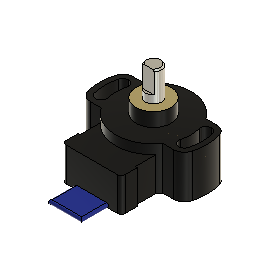
Gas Pedal Sensor Adapter (Autodesk Fusion 360 archive; units mm, degrees)
design "Rotary Hall Effect Pedal Sensor PSC360G2-F2AA-C0002-ERA360-05K"
Autodesk Fusion 360 part; units mm, degrees
note: some values were not read from the file. Chosen so that the rebuilt part matches the saved one: which face or edge a step refers to; that a step has no effect. Set by a fixed rule: which sketch regions a step uses.
sketch "Sketch1" plane through (0, 0, 0) normal (0, 0, 1) x (1, 0, 0)
  circle A0 centre (0, 0) radius 16 construction
  circle A1 centre (0, 0) radius 14
  dimension "d1" = 32
  dimension "d2" = 28
  constraint coincident A0.centre A1.centre
  measures "d1" diameter of A0
  measures "d2" diameter of A1
extrude "Extrude1" add sketch "Sketch1" along normal blind 16
sketch "Sketch2" plane through (0, 0, 0) normal (0, 0, 1) x (1, 0, 0)
  line L0 (0, 0) -> (0, -17) construction
  circle A0 centre (0, 0) radius 14 construction
  line L1 (0, 14) -> (0, -23) construction
  line L2 (0, -23) -> (-11, -23) construction
  line L3 (-11, -23) -> (11, -23)
  line L4 (11, -23) -> (11, -17)
  line L5 (11, -6.2827) -> (-11, -6.2827)
  line L6 (-10.3, -17) -> (-11, -17)
  line L7 (-10.3, -17) -> (-10.3, -4.6882)
  line L8 (-11, -6.2827) -> (-11, -8.6603)
  line L9 (-11, -17) -> (-11, -23)
  line L10 (0, -17) -> (10.3, -17) construction
  line L11 (10.3, -17) -> (11, -17)
  line L12 (10.3, -17) -> (10.3, -1.724)
  dimension "d5" = 17
  dimension "d6" = 37
  dimension "d7" = 11
  dimension "d8" = 22
  dimension "d9" = 10.3
  dimension "d10" = 10.3
  constraint coincident L0.start A0.centre
  constraint vertical L0
  constraint coincident A0 L1.start
  constraint parallel L0 L1
  constraint perpendicular L1 L2
  constraint horizontal L3
  constraint vertical L4
  constraint horizontal L5
  constraint vertical L8
  constraint coincident L6.end L8
  constraint perpendicular L6 L8
  constraint perpendicular L5 L7
  constraint coincident A0 L8.end
  constraint collinear L8 L9
  constraint perpendicular L4 L10
  constraint perpendicular L4 L11
  constraint perpendicular L5 L12
  measures "d5" distance of L0.start L0.end
  measures "d6" distance of L1.start L1.end
  measures "d7" distance of L1.end L2.end
  measures "d8" distance of L2.end L3.end
  measures "d9" distance of L0.end L6.start
  measures "d10" distance of L0.end L10.end
extrude "Extrude2" add sketch "Sketch2" along normal blind 12.5
sketch "Sketch3" plane through (0, 0, 0) normal (0, 0, 1) x (1, 0, 0)
  circle A0 centre (0, 0) radius 20
  line L0 (26.1704, -8) -> (-26.1704, -8)
  line L1 (-26.1704, -8) -> (-26.1704, 8)
  line L2 (-26.1704, 8) -> (26.1704, 8)
  line L3 (26.1704, 8) -> (26.1704, -8)
  line L4 (26.1704, -8) -> (-26.1704, 8) construction
  line L5 (-26.1704, -8) -> (26.1704, 8) construction
  dimension "d13" = 40
  dimension "d14" = 16
  constraint coincident A0.centre origin
  constraint horizontal L0
  constraint perpendicular L0 L1
  constraint parallel L0 L2
  constraint parallel L1 L3
  constraint coincident L4 A0.centre
  constraint coincident L5 A0.centre
  measures "d13" diameter of A0
  measures "d14" distance of L0.end L1.end
extrude "Extrude3" add sketch "Sketch3" along normal blind 16 contours A0 L0 L2
sketch "Sketch4" plane through (0, 0, 0) normal (0, 0, 1) x (1, 0, 0)
  circle A0 centre (-16, 0) radius 2.1
  circle A1 centre (0, 0) radius 16
  circle A2 centre (16, 0) radius 2.1
  circle A3 centre (0, 0) radius 14
  dimension "d17" = 4.2
  dimension "d18" = 4.2
  dimension "d19" = 28
  constraint coincident A0.centre A1
  constraint coincident A1 A2.centre
  constraint concentric A1 A3
  measures "d17" diameter of A0
  measures "d18" diameter of A2
  measures "d19" diameter of A3
extrude "Extrude4" cut sketch "Sketch4" along normal blind 50 contours A0 A3 | A0 A1 A3 | A0 A1 | A2 A3 | A1 A2 A3 | A1 A2
sketch "Sketch5" plane through (0, 0, 16) normal (0, 0, 1) x (-1, 0, 0)
  circle A0 centre (16, 0) radius 2.1
  circle A1 centre (-16, 0) radius 2.1
  arc A2 (11.4891, 8) -> (-11.4891, 8) centre (0, 0) ccw
  line L0 (-11.4891, 8) -> (-18.3303, 8)
  arc A3 (-18.3303, 8) -> (-18.3303, -8) centre (0, 0) ccw
  line L1 (-18.3303, -8) -> (-11.4891, -8)
  arc A4 (-11.4891, -8) -> (11.4891, -8) centre (0, 0) ccw
  line L2 (11.4891, -8) -> (18.3303, -8)
  arc A5 (18.3303, -8) -> (18.3303, 8) centre (0, 0) ccw
  line L3 (18.3303, 8) -> (11.4891, 8)
  line L4 (17.0411, 6.1) -> (10.4499, 6.1)
  arc A6 (10.4499, 6.1) -> (-10.4499, 6.1) centre (0, 0) ccw
  line L5 (-10.4499, 6.1) -> (-17.0411, 6.1)
  arc A7 (-17.0411, 6.1) -> (-17.0411, -6.1) centre (0, 0) ccw
  line L6 (-17.0411, -6.1) -> (-10.4499, -6.1)
  arc A8 (-10.4499, -6.1) -> (10.4499, -6.1) centre (0, 0) ccw
  line L7 (10.4499, -6.1) -> (17.0411, -6.1)
  arc A9 (17.0411, -6.1) -> (17.0411, 6.1) centre (0, 0) ccw
  circle A10 centre (15.4915, -4) radius 2.1
  dimension "d22" = -1.9
  dimension "d23" = 4.2
  dimension "d24" = 2.1
  measures "d23" diameter of A10
  measures "d24" distance of L7 A10.centre
ref_plane "WorkPlane1" through (-14.9097, 0, 8) normal (0, -1, 0) x (1, 0, 0)
extrude "Extrude5" cut sketch "Sketch5" against normal blind 20.219 contours A0 A10 | A0 A10 picked at (15.8466, -1.9917) picked at (15.4687, -4.7533)
mirror "Mirror1" about plane through (-14.9097, 0, 8) normal (0, -1, 0) of "Extrude5"
sketch "Sketch6" plane through (0, 0, 16) normal (0, 0, 1) x (-1, 0, 0)
  arc A0 (16.3288, 2.0741) -> (15.1628, 1.9259) centre (15.4915, 4) ccw
  arc A1 (16.3288, -2.0741) -> (16.3288, 2.0741) centre (16, 0) ccw
  arc A2 (15.1628, -1.9259) -> (16.3288, -2.0741) centre (15.4915, -4) ccw
  arc A3 (15.1628, 1.9259) -> (15.1628, -1.9259) centre (16, 0) ccw
  circle A4 centre (-16, 0) radius 2.1
  arc A5 (11.4891, 8) -> (-11.4891, 8) centre (0, 0) ccw
  line L0 (-11.4891, 8) -> (-18.3303, 8)
  arc A6 (-18.3303, 8) -> (-18.3303, -8) centre (0, 0) ccw
  line L1 (-18.3303, -8) -> (-11.4891, -8)
  arc A7 (-11.4891, -8) -> (11.4891, -8) centre (0, 0) ccw
  line L2 (11.4891, -8) -> (18.3303, -8)
  arc A8 (18.3303, -8) -> (18.3303, 8) centre (0, 0) ccw
  line L3 (18.3303, 8) -> (11.4891, 8)
  circle A9 centre (0, 0) radius 18.0935
  line L4 (17.0402, 6.0832) -> (11.3307, 6.0832)
  line L5 (15.4915, -4) -> (15.5034, -6.1)
  line L6 (17.4872, -6.0832) -> (10.4705, -6.123)
  circle A10 centre (0, 0) radius 13.9
  dimension "d30" = 90
  constraint concentric A5 A9
  constraint coincident A9 L4.start
  constraint horizontal L4
  constraint coincident A2.centre L5.start
  constraint coincident A2 L5.end
  constraint concentric A9 A10
  constraint tangent A3 A10
  measures "d30" angle of L5 L6
extrude "Extrude6" cut sketch "Sketch6" against normal blind 50 contours A0 A1 A9 | A0 A9 L4 | A1 A2 A9 | A0 L4 A10 | A2 A9 L6 | A0 A3 A10 | A2 A3 A10 | A2 L6 A10
delete_face "DeleteFace1" 1 faces at (-17.5465, 4.4327, 10.6667)
delete_face "DeleteFace2" 1 faces at (-15.3853, 6.0973, 10.6667)
delete_face "DeleteFace3" 1 faces at (-18.0955, 0.1367, 10.6667)
delete_face "DeleteFace4" 1 faces at (-15.3442, -6.0948, 5.3333)
delete_face "DeleteFace5" 1 faces at (-17.5295, -4.5066, 10.6667)
delete_face "DeleteFace6" 1 faces at (-15.5262, -6.0832, 10.6667)
fillet "Fillet1" radius 2.1 4 edges at (-17.0393, 6.0858, 8) (-12.4843, 6.1116, 8) (-12.4982, -6.0832, 8) (-17.0402, -6.0832, 8)
delete_face "DeleteFace7" [no effect]
mirror "Mirror2" about plane through (0, 0, 0) normal (1, 0, 0) of 6 faces at (-17.4233, -4.805, 10.6667) (-18.03, -1.515, 10.6667) (-14.2896, -5.7091, 10.6667) (-13.7624, 1.9509, 5.3333) (-15.1741, 6.0721, 10.6667) (-17.2821, 5.0874, 10.6667)
delete_face "DeleteFace8" 1 faces at (18.0955, 0.1367, 10.6667)
sketch "Sketch7" plane through (0, 0, 16) normal (0, 0, 1) x (-1, 0, 0)
  arc A0 (-17.4755, 4.6884) -> (-17.5201, -4.519) centre (0, 0) ccw
  arc A1 (-15.4974, 6.0832) -> (-17.4755, 4.6884) centre (-15.4974, 3.9832) ccw
  line L0 (-15.4974, 6.0832) -> (-15.4963, 6.0832)
  arc A2 (-13.4624, 3.4604) -> (-15.4963, 6.0832) centre (-15.4963, 3.9832) ccw
  arc A3 (-13.4624, 3.4604) -> (-13.4598, -3.4702) centre (0, 0) ccw
  arc A4 (-15.4985, -6.0945) -> (-13.4598, -3.4702) centre (-15.4934, -3.9945) ccw
  arc A5 (-17.5201, -4.519) -> (-15.4985, -6.0945) centre (-15.4866, -3.9945) ccw
  arc A6 (18.3303, -8) -> (18.3303, 8) centre (0, 0) ccw
  line L1 (18.3303, 8) -> (11.4891, 8)
  arc A7 (11.4891, 8) -> (-11.4891, 8) centre (0, 0) ccw
  line L2 (-11.4891, 8) -> (-18.3303, 8)
  arc A8 (-18.3303, 8) -> (-18.3303, -8) centre (0, 0) ccw
  line L3 (-18.3303, -8) -> (-11.4891, -8)
  arc A9 (-11.4891, -8) -> (11.4891, -8) centre (0, 0) ccw
  line L4 (11.4891, -8) -> (18.3303, -8)
  arc A10 (17.4755, 4.6884) -> (15.4974, 6.0832) centre (15.4974, 3.9832) ccw
  arc A11 (17.5201, -4.519) -> (17.4755, 4.6884) centre (0, 0) ccw
  arc A12 (15.4985, -6.0945) -> (17.5201, -4.519) centre (15.4866, -3.9945) ccw
  arc A13 (13.4598, -3.4702) -> (15.4985, -6.0945) centre (15.4934, -3.9945) ccw
  arc A14 (13.4598, -3.4702) -> (13.4624, 3.4604) centre (0, 0) ccw
  arc A15 (15.4963, 6.0832) -> (13.4624, 3.4604) centre (15.4963, 3.9832) ccw
  line L5 (15.4963, 6.0832) -> (15.4974, 6.0832)
  circle A16 centre (0, 0) radius 6.5
  dimension "d37" = 13
  constraint concentric A0 A16
  measures "d37" diameter of A16
extrude "Extrude7" add sketch "Sketch7" along normal blind 5.1 contours A16
sketch "Sketch8" plane through (0, 0, 21.1) normal (0, 0, 1) x (-1, 0, 0)
  circle A0 centre (0, 0) radius 6.5
  circle A1 centre (0, 0) radius 3
  dimension "d40" = 6
  constraint coincident A0.centre A1.centre
  measures "d40" diameter of A1
extrude "Extrude8" add sketch "Sketch8" along normal blind 9.9 contours A1
sketch "Sketch9" plane through (0, 0, 31) normal (0, 0, 1) x (-1, 0, 0)
  circle A0 centre (0, 0) radius 3
  line L0 (0, 0) -> (0.0009, -3) construction
  line L1 (0.0009, -3) -> (-0.0006, 2) construction
  line L2 (3.0076, 2) -> (-4.3795, 1.9979) construction
  line L3 (2.2363, 1.9998) -> (-3.6797, 1.9981)
  dimension "d43" = 5
  constraint coincident A0.centre L0.start
  constraint coincident A0 L0.end
  constraint parallel L0 L1
  constraint perpendicular L1 L2
  constraint coincident L2 L3.start
  constraint coincident A0 L3.start
  constraint coincident L2 L3.end
  constraint perpendicular L1 L3
  measures "d43" distance of L0.end L1.end
extrude "Extrude9" cut sketch "Sketch9" against normal blind 8 contours A0 L3 picked at (0.0625, 2.4741)
extrude "Extrude10" add 1 faces at (-0.7146, 0.4907, 31) along direction (0, 0, 1) blind 1
extrude "Extrude11" add 1 faces at (-0.0625, -2.4741, 23) along direction (0, 0, 1) blind 1
chamfer "Chamfer1" distance 0.5 angle 45 1 edges at (-0.0009, 3, 32)
fillet "Fillet2" radius 4 4 edges at (-18.3303, -8, 8) (-18.3303, 8, 8) (18.3303, -8, 8) (18.3303, 8, 8)
fillet "Fillet3" radius 1.5 2 edges at (11, -23, 6.25) (-11, -23, 6.25)
sketch "Sketch10" plane through (0, -23, 0) normal (0, -1, 0) x (1, 0, 0)
  line L0 (-9.5, 12.5) -> (-9.5, 0)
  line L1 (-9.5, 0) -> (9.5, 0)
  line L2 (9.5, 0) -> (9.5, 12.5)
  line L3 (9.5, 12.5) -> (-9.5, 12.5)
  line L4 (6.25, -1.5) -> (-6.25, -1.5)
  line L5 (-6.25, -1.5) -> (-6.25, 1.5)
  line L6 (-6.25, 1.5) -> (6.25, 1.5)
  line L7 (6.25, 1.5) -> (6.25, -1.5)
  line L8 (6.25, -1.5) -> (-6.25, 1.5) construction
  line L9 (-6.25, -1.5) -> (6.25, 1.5) construction
  dimension "d55" = 12.5
  dimension "d56" = 3
  constraint horizontal L4
  constraint perpendicular L4 L5
  constraint parallel L4 L6
  constraint parallel L5 L7
  constraint coincident L8 origin
  constraint coincident L9 origin
  measures "d55" distance of L5.end L6.end
  measures "d56" distance of L4.end L5.end
extrude "Extrude12" add sketch "Sketch10" along normal blind 10 contours L1 L5 L6 L7
fillet "Fillet4" radius 0.75 6 edges at (0, -33, 1.5) (-6.25, -28, 1.5) (6.25, -28, 1.5) (6.25, -28, 0) (0, -33, 0) (-6.25, -28, 0)
equation "d9 = ( 20.6 / 2 ) * 1 mm"
equation "d10 = ( 20.6 / 2 ) * 1 mm"
equation "d24 = ( 4.2 / 2 ) * 1 mm"
equation "d38 = 21.1 mm - 16 mm"
equation "d41 = 31 mm - 21.1 mm"
